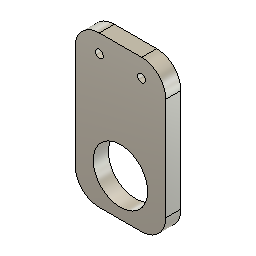
Robot+light+24 (Autodesk Fusion 360 design; units mm, degrees)
Autodesk Fusion 360 part; units mm, degrees
sketch "Sketch1" plane through (0, 0, 0) normal (0, 0, 1) x (1, 0, 0)
  line L0 (10.16, 0) -> (27.94, 0)
  line L1 (38.1, 10.16) -> (38.1, 53.34)
  line L2 (27.94, 63.5) -> (10.16, 63.5)
  line L3 (0, 53.34) -> (0, 10.16)
  circle A0 centre (19.05, 15.875) radius 11.43
  arc A1 (10.16, 63.5) -> (0, 53.34) centre (10.16, 53.34) ccw
  arc A2 (38.1, 53.34) -> (27.94, 63.5) centre (27.94, 53.34) ccw
  arc A3 (27.94, 0) -> (38.1, 10.16) centre (27.94, 10.16) ccw
  arc A4 (0, 10.16) -> (10.16, 0) centre (10.16, 10.16) ccw
  circle A5 centre (10.16, 55.88) radius 1.651
  line L4 (19.05, 63.5) -> (19.05, 0) construction
  circle A6 centre (27.94, 55.88) radius 1.651
  point P0 (38.1, 0)
  point P1 (0, 63.5)
  dimension "d1" = 38.1
  dimension "d2" = 63.5
  dimension "d3" = 22.86
  dimension "d4" = 10.16
  dimension "d5" = 3.302
  dimension "d6" = 7.62
  dimension "d7" = 10.16
  dimension "d8" = 19.05
  dimension "d9" = 15.875
  constraint horizontal L0
  constraint vertical L1
  constraint horizontal L2
  constraint vertical L3
  constraint coincident P1 L3
  constraint coincident P1 L2
  constraint tangent L3 A1
  constraint tangent L2 A1
  constraint tangent L2 A2
  constraint tangent L1 A2
  constraint equal A1 A2
  constraint coincident P0 L1
  constraint coincident P0 L0
  constraint tangent L1 A3
  constraint tangent L0 A3
  constraint equal A1 A3
  constraint coincident origin L3
  constraint coincident origin L0
  constraint tangent L3 A4
  constraint tangent L0 A4
  constraint equal A1 A4
  constraint midpoint L2 L4.start
  constraint midpoint L0 L4.end
  constraint symmetric A5 L4 A6
  measures "d1" distance of origin P0
  measures "d2" distance of origin P1
  measures "d3" diameter of A0
  measures "d4" radius of A1
  measures "d5" diameter of A5
  measures "d6" distance of L2 A5.centre
  measures "d7" distance of L3 A5.centre
  measures "d8" distance of L1 A0.centre
  measures "d9" distance of A0.centre L4.end
extrude "Extrude1" add sketch "Sketch1" along normal blind 6.35
